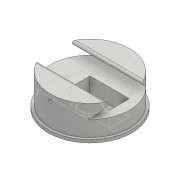
# Autodesk Inventor part: arm_0_top
Saved by Autodesk Inventor 2018 (Build 220112000, 112)
## iProperties
Created: 2017-12-03
Part Number: arm_0_top
Material: Generic
Document SubType Name: Modeling
Designer: Bardo91
Density: 1 g/cm^3
Appearance: Default
Author: Bardo91
Autodesk Inventor part; units mm, degrees
ref_plane "YZ Plane" through (0, 0, 0) normal (1, 0, 0) x (0, 1, 0)
ref_plane "XZ Plane" through (0, 0, 0) normal (0, 1, 0) x (-1, 0, 0)
ref_plane "XY Plane" through (0, 0, 0) normal (0, 0, 1) x (1, 0, 0)
sketch "Sketch1" plane through (0, 0, 0) normal (0, 0, 1) x (1, 0, 0)
  circle A0 centre (0, 0) radius 40
  dimension "d0" = 80
  constraints: 1 centre point, 1 coincident
  measures "d0" diameter of A0
extrude "base" add sketch "Sketch1" along normal blind 30
sketch "Sketch3" plane through (0, 0, 0) normal (1, 0, 0) x (0, 1, 0)
  line L0 (40, 30) -> (-40, 30) projected
  line L1 (0, 30) -> (-15, 30)
  line L2 (0, 30) -> (15, 30)
  line L3 (15, 30) -> (29.1421, 15.8579)
  line L4 (-15, 30) -> (-29.1421, 15.8579)
  line L5 (-15, 30) -> (5, 30) construction
  line L6 (-29.1421, 15.8579) -> (29.1421, 15.8579)
  point P0 (0, 0)
  dimension "d13" = 15
  dimension "d14" = 15
  dimension "d15" = 20
  dimension "d16" = 135
  dimension "d17" = 20
  dimension "d18" = 135
  constraints: 12 end point, 2 point on line, 1 equal length, 1 horizontal, 1 midpoint
  measures "d13" distance of L1.start L1.end
  measures "d14" distance of L1.start L2.end
  measures "d15" distance of L2.end L3.end
  measures "d16" angle of L2 L3
  measures "d17" distance of L1.end L4.end
  measures "d18" angle of L4 L5
extrude "horse_tail_1" cut sketch "Sketch3" against normal up to surface round surface about axis through (0, 0, 0) along (0, 0, 1) radius 40 far side no
mirror "horse_tail_2" about plane through (0, 0, 21.3699) normal (-1, 0, 0) of "horse_tail_1"
fillet "fillet_horse_tail" radius 2 2 edges at (0, 15, 30) (0, -15, 30)
sketch "Sketch4" plane through (0, 0, 0) normal (0, 1, 0) x (-1, 0, 0)
  line L0 (34.7395, 30) -> (-34.7395, 30) projected
  circle A0 centre (0, 23.8579) radius 1.75
  line L1 (0, 23.8579) -> (0, 15.8579)
  line L2 (-27.3996, 15.8579) -> (27.3996, 15.8579) projected
  point P0 (0, 0)
  dimension "d20" = 3.5
  dimension "d23" = 8
  constraints: 2 end point, 1 centre point, 1 midpoint
  measures "d20" diameter of A0
  measures "d23" distance of L1.start L1.end
extrude "lock_arm" cut sketch "Sketch4" along normal through all both and the other way through all
sketch "Sketch5" plane through (-27.3996, -29.1421, 15.8579) normal (0, 0, 1) x (1, 0, 0)
  line L0 (27.3996, 29.1421) -> (27.3996, 19.1421)
  line L1 (27.3996, 19.1421) -> (17.3996, 19.1421)
  line L2 (17.3996, 19.1421) -> (17.3996, 39.1421)
  line L3 (17.3996, 39.1421) -> (57.3996, 39.1421)
  line L4 (57.3996, 39.1421) -> (57.3996, 19.1421)
  line L5 (57.3996, 19.1421) -> (27.3996, 19.1421)
  dimension "d24" = 10
  dimension "d25" = 10
  dimension "d26" = 20
  dimension "d27" = 40
  constraints: 12 end point, 5 perpendicular, 1 point on line, 1 vertical
  measures "d24" distance of L0.start L0.end
  measures "d25" distance of L0.end L1.end
  measures "d26" distance of L1.end L2.end
  measures "d27" distance of L2.end L3.end
extrude "servo_place" cut sketch "Sketch5" against normal through all
sketch "Sketch6" plane through (0, 0, 0) normal (0, 0, -1) x (-1, 0, 0)
  circle A0 centre (0, 0) radius 10
  circle A1 centre (0, 0) radius 42.5
  dimension "d30" = 20
  dimension "d31" = 85
  constraints: 2 centre point, 2 coincident
  measures "d30" diameter of A0
  measures "d31" diameter of A1
extrude "base_hold" add sketch "Sketch6" along normal blind 3
body "Solid1"
